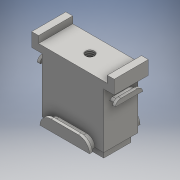
# Autodesk Inventor part: Sample-cuvette-clamp-20mm-V4
Saved by Autodesk Inventor 2016 (Build 200138000, 138)
## iProperties
Created: 2018-06-04
Part Number: Sample-cuvette-clamp-20mm-V4
Material: Generic
Document SubType Name: Modeling
Designer: voigt
Density: 1 g/cm^3
Appearance: Default
Author: voigt
Autodesk Inventor part; units mm, degrees
ref_plane "YZ Plane" through (0, 0, 0) normal (1, 0, 0) x (0, 1, 0)
sketch "Sketch1" plane through (0, 0, 0) normal (0, 0, 1) x (1, 0, 0)
  line L0 (0, 6.93) -> (0, -6.93) construction
  line L1 (-13.93, 0) -> (13.93, 0) construction
  line L2 (-9.95, 4.95) -> (9.95, 4.95)
  line L3 (9.95, 4.95) -> (9.95, -4.95)
  line L4 (9.95, -4.95) -> (-9.95, -4.95)
  line L5 (-9.95, -4.95) -> (-9.95, 4.95)
  point P0 (0, 0)
  dimension "d0" = 9.9
  dimension "d1" = 19.9
  constraints: 8 end point, 2 parallel, 1 horizontal, 1 perpendicular, 2 other
  measures "d0" distance between parallel lines of L4 L2
  measures "d1" distance between parallel lines of L3 L5
extrude "Extrusion1" add sketch "Sketch1" along normal blind 3
sketch "Sketch2" plane through (0, 0, 3) normal (0, 0, 1) x (1, 0, 0)
  line L0 (9.95, 4.95) -> (-9.95, 4.95) construction
  line L1 (-9.95, 4.95) -> (-9.95, -4.95) construction
  line L2 (-9.95, -4.95) -> (9.95, -4.95) construction
  line L3 (9.95, -4.95) -> (9.95, 4.95) construction
  line L4 (11.2, 6.2) -> (-11.2, 6.2)
  line L5 (-11.2, 6.2) -> (-11.2, -6.2)
  line L6 (-11.2, -6.2) -> (11.2, -6.2)
  line L7 (11.2, -6.2) -> (11.2, 6.2)
  point P0 (0, 0)
  dimension "d" = 1.25
  dimension "d5" = 1.25
  dimension "d6" = 1.25
  dimension "d7" = 1.25
  constraints: 8 end point, 2 parallel, 1 horizontal, 1 perpendicular
  measures "d" distance between parallel lines of L3 L7
  measures "d5" distance between parallel lines of L0 L4
  measures "d6" distance between parallel lines of L5 L1
  measures "d7" distance between parallel lines of L6 L2
extrude "Extrusion2" add sketch "Sketch2" along normal blind 20
sketch "Sketch3" plane through (0, 0, 23) normal (0, 0, 1) x (1, 0, 0)
  line L0 (11.2, 6.2) -> (-11.2, 6.2) construction
  line L1 (-11.2, 6.2) -> (-11.2, -6.2) construction
  line L2 (-11.2, -6.2) -> (11.2, -6.2) construction
  line L3 (11.2, -6.2) -> (11.2, 6.2) construction
  line L4 (0, 8.68) -> (0, -8.68) construction
  line L5 (-21, 0) -> (21, 0) construction
  line L6 (15, 6.2) -> (-15, 6.2)
  line L7 (-15, 6.2) -> (-15, -6.2)
  line L8 (-15, -6.2) -> (15, -6.2)
  line L9 (15, -6.2) -> (15, 6.2)
  point P0 (0, 0)
  dimension "d10" = 30
  constraints: 8 end point, 2 collinear, 2 parallel, 1 horizontal, 1 perpendicular, 1 other
  measures "d10" distance between parallel lines of L7 L9
extrude "Extrusion3" add sketch "Sketch3" along normal blind 5
sketch "Sketch4" plane through (0, 0, 28) normal (0, 0, 1) x (1, 0, 0)
  line L0 (0, 17.5) -> (0, -17.5) construction
  line L1 (-21, 0) -> (21, 0) construction
  line L2 (15, 6.2) -> (-15, 6.2) construction
  line L3 (-15, 6.2) -> (-15, -6.2) construction
  line L4 (-15, -6.2) -> (15, -6.2) construction
  line L5 (15, -6.2) -> (15, 6.2) construction
  line L6 (12.5, 12.5) -> (-12.5, 12.5)
  line L7 (-12.5, 12.5) -> (-12.5, -12.5)
  line L8 (-12.5, -12.5) -> (12.5, -12.5)
  line L9 (12.5, -12.5) -> (12.5, 12.5)
  point P0 (0, 0)
  dimension "d13" = 25
  dimension "d14" = 25
  constraints: 8 end point, 2 parallel, 1 horizontal, 1 perpendicular, 2 other
  measures "d13" distance between parallel lines of L7 L9
  measures "d14" distance of L8.end L6.start
extrude "Extrusion4" cut sketch "Sketch4" against normal blind 2.5
sketch "Sketch5" plane through (0, 0, 25.5) normal (0, 0, 1) x (1, 0, 0)
  point P0 (0, 0)
  point P1 (0, 0)
  constraints: 1 coincident
hole "Hole1" at (0, 0, 25.5) direction (0, 0, -1) diameter 3.242 depth 10 tip angle 118 thread size "M4x0.7" class "6H" standard "ANSI Metric M Profile"
sketch "Sketch6" plane through (-11.2, -6.2, 3) normal (0, -1, 0) x (1, 0, 0)
  line L0 (-1.3, 22.5) -> (-1.3, 25) construction
  line L1 (-3.8, 25) -> (-1.3, 25) construction
  line L2 (-3.8, 20) -> (-3.8, 25) construction
  line L3 (-3.8, 20) -> (0, 20) construction
  line L4 (0, 0) -> (0, 20) construction
  line L5 (0, 0) -> (22.4, 0) construction
  line L6 (22.4, 0) -> (22.4, 20) construction
  line L7 (22.4, 20) -> (26.2, 20) construction
  line L8 (26.2, 20) -> (26.2, 25) construction
  line L9 (23.7, 25) -> (26.2, 25) construction
  line L10 (23.7, 25) -> (23.7, 22.5) construction
  line L11 (23.7, 22.5) -> (-1.3, 22.5) construction
  line L12 (11.2, 30.6) -> (11.2, -8.6) construction
  line L13 (0, 0) -> (22.4, 0) projected
  line L14 (3.2, 0) -> (11.2, 0)
  arc A0 (6.2, 3) -> (3.2, 0) centre (6.2, 0) ccw
  line L15 (6.2, 3) -> (11.2, 3)
  line L16 (19.2, 0) -> (11.2, 0)
  arc A1 (19.2, 0) -> (16.2, 3) centre (16.2, 0) ccw
  line L17 (16.2, 3) -> (11.2, 3)
  point P0 (11.2, -3)
  dimension "d24" = 8
  dimension "r" = 3
  dimension "d28" = 3
  constraints: 8 end point, 4 point on circle, 4 point on line, 3 symmetric about line, 2 centre point, 1 horizontal, 1 midpoint, 1 other
  measures "d24" distance of L14.end L14.start
  measures "r" distance of L14.start A0.centre
  measures "d28" distance between parallel lines of L14 L15
extrude "Extrusion5" add sketch "Sketch6" along normal blind 2
sketch "Sketch7" plane through (-11.2, -8.2, 3) normal (0, -1, 0) x (1, 0, 0)
  line L0 (3.2, 0) -> (19.2, 0) construction
  arc A0 (19.2, 0) -> (16.2, 3) centre (16.2, 0) ccw construction
  line L1 (16.2, 3) -> (6.2, 3) construction
  arc A1 (6.2, 3) -> (3.2, 0) centre (6.2, 0) ccw construction
  line L2 (2.2, 0) -> (20.2, 0) construction
  arc A2 (6.2, 4) -> (2.2, 0) centre (6.2, 0) ccw
  arc A3 (20.2, 0) -> (16.2, 4) centre (16.2, 0) ccw
  line L3 (6.2, 4) -> (16.2, 4)
  line L4 (2.2, 0) -> (20.2, 0)
  point P0 (11.2, -3)
  dimension "d33" = 1
  dimension "a" = 1
  constraints: 6 end point, 4 point on circle, 2 centre point, 2 coincident, 1 collinear, 1 horizontal, 1 tangent
  measures "d33" distance of L0.start L2.start
  measures "a" distance of L2.end L0.end
extrude "Extrusion6" add sketch "Sketch7" along normal blind 1
ref_plane "Work Plane1" through (11.2, 0, 23) normal (0, -1, 0) x (1, 0, 0)
ref_plane "Work Plane2" through (0, -6.2, 3) normal (-1, 0, 0) x (0, 0, 1)
mirror "Mirror1" about plane through (11.2, 0, 23) normal (0, -1, 0) of "Extrusion5", "Extrusion6"
sketch "Sketch8" plane through (-11.2, -6.2, 3) normal (-1, 0, 0) x (0, 0, 1)
  line L0 (0, 12.4) -> (0, 0) construction
  line L1 (0, 0) -> (20, 0) construction
  line L2 (20, 12.4) -> (20, 0) construction
  line L3 (0, 12.4) -> (20, 12.4) construction
  line L4 (30.6, 6.2) -> (-8.6, 6.2) construction
  line L5 (15, 10.2) -> (15, 6.2)
  arc A0 (16, 9.2) -> (15, 10.2) centre (15, 9.2) ccw
  line L6 (15, 9.2) -> (16, 9.2) construction
  line L7 (15, 9.2) -> (15, 10.2) construction
  line L8 (16, 9.2) -> (16, 6.2)
  line L9 (15, 2.2) -> (15, 6.2)
  arc A1 (15, 2.2) -> (16, 3.2) centre (15, 3.2) ccw
  line L10 (16, 3.2) -> (16, 6.2)
  point P0 (-3, 6.2)
  dimension "d37" = 4
  dimension "d38" = 90
  dimension "radius" = 1
  dimension "d40" = 15
  constraints: 12 end point, 4 point on circle, 4 point on line, 3 symmetric about line, 2 centre point, 2 perpendicular, 1 other
  measures "d37" distance from line of L4 L5.start
  measures "d38" angle of L6 L7
  measures "radius" radius of A0
  measures "d40" distance between parallel lines of L0 L5
extrude "Extrusion7" add sketch "Sketch8" along normal blind 2
sketch "Sketch9" plane through (-13.2, -6.2, 3) normal (-1, 0, 0) x (0, 0, 1)
  line L0 (15, 10.2) -> (15, 2.2) construction
  arc A0 (15, 2.2) -> (16, 3.2) centre (15, 3.2) ccw construction
  line L1 (16, 3.2) -> (16, 9.2) construction
  arc A1 (16, 9.2) -> (15, 10.2) centre (15, 9.2) ccw construction
  line L2 (15, 11.2) -> (15, 1.2)
  arc A2 (17, 9.2) -> (15, 11.2) centre (15, 9.2) ccw
  arc A3 (15, 1.2) -> (17, 3.2) centre (15, 3.2) ccw
  line L3 (17, 9.2) -> (17, 3.2)
  line L4 (15, 10.2) -> (15, 2.2) projected
  point P0 (-3, 6.2)
  dimension "d44" = 1
  dimension "d45" = 1
  dimension "d46" = 90
  constraints: 4 end point, 4 point on circle, 2 centre point, 2 coincident, 2 vertical, 1 collinear
  measures "d44" distance of L0.start L2.start
  measures "d45" distance of L2.end L0.end
extrude "Extrusion8" add sketch "Sketch9" along normal blind 1
fillet "Fillet1" radius 0.25 5 edges at (-12.2, 4, 18) (-13.7, 5, 18) (-13.7, -5, 18) (-12.2, -4, 18) (-14.2, 0, 18)
mirror "Mirror2" about plane through (0, -6.2, 3) normal (-1, 0, 0) of "Extrusion7", "Extrusion8", "Fillet1"
equation "\"d5\" = d"
equation "\"d6\" = d"
equation "\"d7\" = d"
equation "\"d28\" = r"
equation "\"d33\" = a"
body "Solid1"
